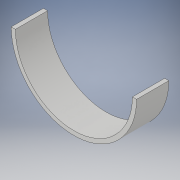
# Autodesk Inventor part: BallPath180
Saved by Autodesk Inventor 2017 (Build 210142000, 142)
## iProperties
Created: 2016-09-18
Part Number: BallPath180
Material: Generic
Document SubType Name: Modeling
Designer: Spartacles
Density: 1 g/cm^3
Appearance: Default
Author: Spartacles
Autodesk Inventor part; units mm, degrees
ref_plane "YZ Plane" through (0, 0, 0) normal (1, 0, 0) x (0, 1, 0)
ref_plane "XZ Plane" through (0, 0, 0) normal (0, 1, 0) x (-1, 0, 0)
ref_plane "XY Plane" through (0, 0, 0) normal (0, 0, 1) x (1, 0, 0)
sketch "Sketch2" plane through (0, 0, 0) normal (0, 1, 0) x (-1, 0, 0)
  line L0 (0, 0) -> (12.7, 0)
  line L1 (12.7, 0) -> (12.7, -97.79)
  line L2 (12.7, -97.79) -> (0, -97.79)
  line L3 (0, -97.79) -> (0, 0)
  line L4 (368.3, 0) -> (381, 0)
  line L5 (381, 0) -> (381, -97.79)
  line L6 (381, -97.79) -> (368.3, -97.79)
  line L7 (368.3, -97.79) -> (368.3, 0)
  dimension "d0" = 12.7
  dimension "d1" = 97.79
  dimension "d2" = 12.7
  dimension "d3" = 97.79
  constraints: 16 end point, 4 parallel, 2 horizontal, 2 perpendicular, 1 point on line
  measures "d0" distance of L1.end L2.end
  measures "d1" distance of L0.end L1.end
  measures "d2" distance of L6.end L5.end
  measures "d3" distance of L4.end L5.end
sketch "Sketch3" plane through (0, 0, 0) normal (0, 0, 1) x (1, 0, 0)
  arc A0 (-368.3, 0) -> (-12.7, 0) centre (-190.5, 0) ccw
  point P0 (0, 0)
  constraints: 2 point on circle, 1 centre point
sweep "Sweep1" add profiles "Sketch2" path "Sketch3"
equation "\"d1\" = d3"
body "Solid1"
